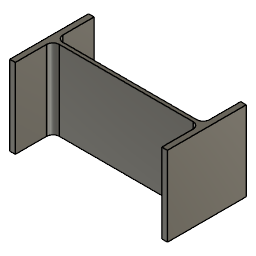
H-198×99×4.5×7 (Autodesk Fusion 360 design; units mm, degrees)
Autodesk Fusion 360 part; units mm, degrees
sketch "スケッチ1" plane through (0, 0, 0) normal (0, 0, 1) x (1, 0, 0)
  line L0 (183, 2.25) -> (15, 2.25)
  line L1 (15, -2.25) -> (183, -2.25)
  line L2 (0, 49.5) -> (0, -49.5)
  line L3 (7, 10.25) -> (7, 49.5)
  line L4 (7, -49.5) -> (7, -10.25)
  line L5 (0, -49.5) -> (7, -49.5)
  line L6 (7, 49.5) -> (0, 49.5)
  line L7 (191, 49.5) -> (191, 10.25)
  line L8 (198, -49.5) -> (198, 49.5)
  line L9 (191, -10.25) -> (191, -49.5)
  line L10 (191, -49.5) -> (198, -49.5)
  line L11 (198, 49.5) -> (191, 49.5)
  arc A0 (15, -2.25) -> (7, -10.25) centre (15, -10.25) ccw
  arc A1 (7, 10.25) -> (15, 2.25) centre (15, 10.25) ccw
  arc A2 (183, 2.25) -> (191, 10.25) centre (183, 10.25) ccw
  arc A3 (191, -10.25) -> (183, -2.25) centre (183, -10.25) ccw
extrude "押し出し1" add sketch "スケッチ1" along normal blind 100
